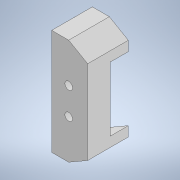
# Autodesk Inventor part: Home Switch Mount X
Saved by Autodesk Inventor 2022 (Build 260153000, 153)
## iProperties
Created: 2021-11-21
Part Number: Home Switch Mount X
Material: Generic
Document SubType Name: Modeling
Designer: nicol
Density: 1 g/cm^3
Appearance: Default
Author: nicol
Autodesk Inventor part; units mm, degrees
ref_plane "YZ Plane" through (0, 0, 0) normal (1, 0, 0) x (0, 1, 0)
ref_plane "XZ Plane" through (0, 0, 0) normal (0, 1, 0) x (-1, 0, 0)
ref_plane "XY Plane" through (0, 0, 0) normal (0, 0, 1) x (1, 0, 0)
sketch "Sketch1" plane through (0, 0, 0) normal (0, 0, 1) x (1, 0, 0)
  line L0 (12.7, 0) -> (12.7, 5.5)
  line L1 (0, 0) -> (12.7, 0)
  line L2 (12.7, 0) -> (12.7, 37.3027)
  line L3 (12.7, 37.3027) -> (0, 37.3027)
  line L4 (0, 37.3027) -> (0, 0)
  line L5 (6, 37.3027) -> (12.7, 33.4345)
  line L6 (6, 0) -> (12.7, 3.8682)
  circle A0 centre (6, 13.9014) radius 1.35
  circle A1 centre (6, 23.4014) radius 1.35
  line L7 (6, 23.4014) -> (6, 13.9014) construction
  line L8 (0, 0) -> (12.7, 7.3323)
  line L9 (12.7, 29.9704) -> (0, 37.3027)
  point P0 (6, 18.6514)
  point P1 (12.7, 18.6514)
  point P2 (12.7, 0)
  dimension "d2" = 9.5
  dimension "d3" = 2.7
  dimension "d4" = 2.7
  dimension "d15" = 37.3027
  dimension "d17" = 60
  dimension "d18" = 60
  dimension "d19" = 3
  dimension "d20" = 3
  dimension "d21" = 12.7
  constraints: 20 end point, 6 point on line, 2 centre point, 2 midpoint, 2 parallel, 1 coincident, 1 collinear, 1 horizontal, 1 horizontal alignment, 1 perpendicular, 1 vertical, 1 vertical alignment
  measures "d2" distance of L7.end L7.start
  measures "d3" diameter of A1
  measures "d4" diameter of A0
  measures "d15" distance of L3.end L1.start
  measures "d17" angle of L4 L8
  measures "d18" angle of L4 L9
  measures "d19" distance between parallel lines of L5 L9
  measures "d20" distance between parallel lines of L6 L8
  measures "d21" distance of L2.end L3.end
extrude "Extrusion1" add sketch "Sketch1" along normal blind 8 contours L6 L1 L8 L2 L0 | L4 L9 L2 L8 | L3 L5 L2 L9
extrude "Extrusion2" add sketch "Sketch1" against normal blind 6.35 contours L6 L1 L8 L2 L0 | L3 L5 L2 L9
equation "\"d4\" = d3"
body "Solid1"
